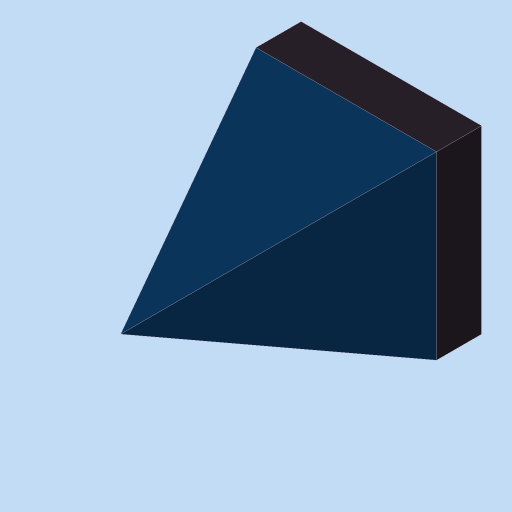
# Autodesk Inventor part: Absorber - SEA-PM5
Saved by Autodesk Inventor 2023.2 (Build 272271000, 271)
## iProperties
Created: 2023-11-29
Part Number: Absorber - SEA-PM5
Material: Generisch
Document SubType Name: Modeling
Designer: Nils Bade
Density: 1 g/cm^3
Appearance: DIY Schwarz
Author: Nils Bade
Autodesk Inventor part; units mm, degrees
ref_plane "YZ Plane" through (0, 0, 0) normal (1, 0, 0) x (0, 1, 0)
ref_plane "XZ Plane" through (0, 0, 0) normal (0, 1, 0) x (-1, 0, 0)
ref_plane "XY Plane" through (0, 0, 0) normal (0, 0, 1) x (1, 0, 0)
sketch "Absorber-Base" plane through (0, 0, 0) normal (0, 0, 1) x (1, 0, 0)
  line L0 (-20, 20) -> (20, 20)
  line L1 (20, 20) -> (20, -20)
  line L2 (20, -20) -> (-20, -20)
  line L3 (-20, -20) -> (-20, 20)
  line L4 (-20, 20) -> (20, -20) construction
  line L5 (20, 20) -> (-20, -20) construction
  point P0 (0, 0)
  dimension "d0" = 40
  constraints: 12 end point, 2 midpoint, 2 parallel, 2 perpendicular, 1 horizontal
  measures "d0" distance of L1.end L2.end
extrude "Gesamtvolumen" add sketch "Absorber-Base" along normal blind 60
sketch "Skizze2" plane through (0, 0, 0) normal (0, 1, 0) x (-1, 0, 0)
  line L0 (-28, 0) -> (28, 0) projected
  line L1 (20, 0) -> (20, 60) projected
  line L2 (-20, 0) -> (-20, 60) projected
  line L3 (20, 0) -> (-20, 0)
  line L4 (-20, 0) -> (-20, 10)
  line L5 (-20, 10) -> (20, 10)
  line L6 (20, 10) -> (20, 0)
  line L7 (-20, 60) -> (20, 60) projected
  line L8 (0, 60) -> (20, 10)
  line L9 (0, 60) -> (-20, 10)
  point P0 (0, 0)
  point P1 (20, 10)
  dimension "d6" = 10
  constraints: 12 end point, 2 parallel, 1 horizontal, 1 midpoint, 1 perpendicular, 1 point on line
  measures "d6" distance between parallel lines of L0 L5
extrude "Cutaway" cut sketch "Skizze2" along normal mid plane 40 contours L2 L7 L9 | L8 L7 L1
pattern_circular "Runde Anordnung1" count 2 over 90 about axis through (0, 0, -10) along (0, 0, 1) of "Cutaway"
equation "\"d0\" = Base_Seitenlänge"
equation "\"d1\" = Gesamthöhe"
equation "\"d6\" = Base_Höhe"
equation "\"d7\" = Base_Seitenlänge"
equation "\"Base_Seitenlänge\" = 40"
equation "\"Base_Höhe\" = 10"
equation "\"Gesamthöhe\" = 60"
